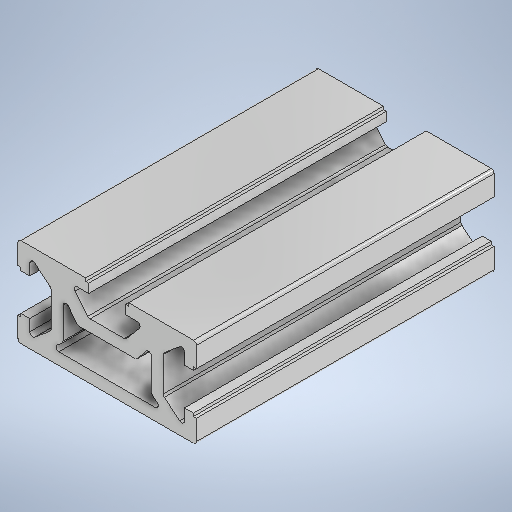
# Autodesk Inventor part: perfil_15x30_001
Saved by Autodesk Inventor 2025.2 (Build 292293000, 293)
## iProperties
Created: 2025-03-25
Part Number: perfil_15x30_001
Material: Alumínio 6061
Document SubType Name: Modeling
Designer: Carlos Dias
Density: 2.7 g/cm^3
Appearance: Alumínio - Polido
Author: Carlos Dias
Autodesk Inventor part; units mm, degrees
ref_plane "YZ Plane" through (0, 0, 0) normal (1, 0, 0) x (0, 1, 0)
ref_plane "XZ Plane" through (0, 0, 0) normal (0, 1, 0) x (-1, 0, 0)
ref_plane "XY Plane" through (0, 0, 0) normal (0, 0, 1) x (1, 0, 0)
sketch "Esboço1" plane through (0, 0, 0) normal (0, 0, 1) x (1, 0, 0)
  line L0 (-15, 15) -> (15, 15) construction
  line L1 (-15, 15) -> (-15, 10.6) construction
  line L2 (-15, 10.6) -> (-13, 10.6) construction
  line L3 (-13, 13.6) -> (-13, 10.6) construction
  line L4 (-13, 13.6) -> (-9.4247, 10.6) construction
  line L5 (-9.4247, 10.6) -> (-9.4247, 4.4) construction
  line L6 (-9.4247, 4.4) -> (-13, 1.4) construction
  line L7 (-13, 4.4) -> (-13, 1.4) construction
  line L8 (-15, 4.4) -> (-13, 4.4) construction
  line L9 (-15, 4.4) -> (-15, 0) construction
  line L10 (-15, 0) -> (0, 0) construction
  line L11 (-15, 4.4) -> (-14.5, 4.4) construction
  line L12 (-14.5, 4.4) -> (-14.5, 3.9)
  line L13 (-14.5, 3.9) -> (-15, 3.9)
  line L14 (-15, 3.9) -> (-15, 4.4) construction
  line L15 (-15, 10.6) -> (-14.5, 10.6) construction
  line L16 (-14.5, 10.6) -> (-14.5, 11.1)
  line L17 (-14.5, 11.1) -> (-15, 11.1)
  line L18 (-15, 11.1) -> (-15, 10.6) construction
  line L19 (-3.1, 9.4247) -> (3.1, 9.4247) construction
  line L20 (-6.1, 13) -> (-3.1, 9.4247) construction
  line L21 (-6.1, 13) -> (-3.1, 13) construction
  line L22 (-3.1, 15) -> (-3.1, 13) construction
  line L23 (-3.1, 9.4247) -> (0, 9.4247) construction
  line L24 (-3.1, 15) -> (-3.6, 15) construction
  line L25 (-3.6, 15) -> (-3.6, 14.5)
  line L26 (-3.6, 14.5) -> (-3.1, 14.5)
  line L27 (-3.1, 14.5) -> (-3.1, 15) construction
  line L28 (-9.4247, 2) -> (0, 2) construction
  line L29 (-7.4247, 3.6782) -> (-9.4247, 2) construction
  line L30 (-7.4247, 10.6) -> (-7.4247, 3.6782) construction
  line L31 (-7.4247, 10.6) -> (-4.944, 7.4247) construction
  line L32 (-4.944, 7.4247) -> (0, 7.4247) construction
  arc A0 (-14.5, 15) -> (-15, 14.5) centre (-14.5, 14.5) ccw
  arc A1 (-12.1786, 12.9108) -> (-13, 12.5277) centre (-12.5, 12.5277) ccw
  line L33 (-14.5, 15) -> (-3.6, 15)
  line L34 (-13, 12.5277) -> (-13, 10.6)
  line L35 (-13, 10.6) -> (-14.5, 10.6)
  arc A2 (-9.4247, 10.3668) -> (-9.6033, 10.7499) centre (-9.9247, 10.3668) ccw
  arc A3 (-9.6033, 4.2501) -> (-9.4247, 4.6332) centre (-9.9247, 4.6332) ccw
  arc A4 (-13, 2.4723) -> (-12.1786, 2.0892) centre (-12.5, 2.4723) ccw
  line L36 (-12.1786, 12.9108) -> (-9.6033, 10.7499)
  line L37 (-9.4247, 10.3668) -> (-9.4247, 4.6332)
  line L38 (-9.6033, 4.2501) -> (-12.1786, 2.0892)
  line L39 (-13, 2.4723) -> (-13, 4.4)
  arc A5 (-15, 0.5) -> (-14.5, 0) centre (-14.5, 0.5) ccw
  line L40 (-15, 14.5) -> (-15, 11.1)
  line L41 (-15, 3.9) -> (-15, 0.5)
  line L42 (-14.5, 0) -> (0, 0)
  arc A6 (-8.4247, 2.8391) -> (-8.1193, 2) centre (-8.1193, 2.4751) ccw
  arc A7 (-6.5307, 9.4557) -> (-7.4247, 9.1479) centre (-6.9247, 9.1479) ccw
  line L43 (-8.1193, 2) -> (0, 2)
  arc A8 (-7.6033, 3.5283) -> (-7.4247, 3.9114) centre (-7.9247, 3.9114) ccw
  arc A9 (-5.0941, 7.6169) -> (-4.7001, 7.4247) centre (-4.7001, 7.9247) ccw
  arc A10 (-3.2499, 9.6033) -> (-2.8668, 9.4247) centre (-2.8668, 9.9247) ccw
  arc A11 (-5.0277, 13) -> (-5.4108, 12.1786) centre (-5.0277, 12.5) ccw
  line L44 (-5.0277, 13) -> (-3.1, 13)
  line L45 (-5.4108, 12.1786) -> (-3.2499, 9.6033)
  line L46 (-2.8668, 9.4247) -> (0, 9.4247)
  line L47 (-4.7001, 7.4247) -> (0, 7.4247)
  line L48 (-6.5307, 9.4557) -> (-5.0941, 7.6169)
  line L49 (-7.4247, 9.1479) -> (-7.4247, 3.9114)
  line L50 (0, 2) -> (0, 0)
  line L51 (0, 7.4247) -> (0, 9.4247)
  line L52 (-3.1, 14.5) -> (-3.1, 13)
  line L53 (-14.5, 4.4) -> (-13, 4.4)
  line L54 (-8.4247, 2.8391) -> (-7.6033, 3.5283)
  point P0 (0, 0)
  point P1 (0, 15)
  point P2 (-14, 4.4)
  point P3 (-1.55, 9.4247)
  point P4 (-9.6033, 10.7499)
  dimension "d0" = 30
  dimension "d1" = 15
  dimension "d6" = 2
  dimension "d7" = 3
  dimension "d9" = 50
  dimension "d12" = 0.5
  dimension "d18" = 50
  dimension "d19" = 2
  dimension "d21" = 2
  dimension "d22" = 2
  dimension "d24" = 2
  dimension "d25" = 0.5
  dimension "d26" = 0.5
  dimension "d27" = 0.5
  dimension "d28" = 0.5
  dimension "d29" = 0.5
  dimension "d30" = 0.5
  dimension "d31" = 0.5
  dimension "d32" = 0.5
  dimension "d33" = 0.5
  dimension "d34" = 0.5
  dimension "d35" = 0.5
  dimension "d38" = 3.1
  dimension "d39" = 6.2
  dimension "d40" = 15
  constraints: 110 end point, 29 point on line, 27 tangent, 24 point on circle, 16 collinear, 12 centre point, 12 equal length, 12 horizontal, 9 vertical, 7 parallel, 7 vertical alignment, 5 midpoint, 4 perpendicular, 2 horizontal alignment, 1 coincident
  measures "d0" distance of L0.start L0.end
  measures "d1" distance from line of point (0, 0) L0
  measures "d6" distance of L1.end L2.end
  measures "d7" distance of L3.start L2.end
  measures "d9" angle of L4 L3
  measures "d12" distance of L16.end L17.end
  measures "d18" angle of L20 L21
  measures "d19" distance between parallel lines of L10 L28
  measures "d21" distance between parallel lines of L5 L30
  measures "d22" angle of L20 L31
  measures "d24" distance between parallel lines of L19 L32
  measures "d25" radius of A0
  measures "d26" radius of A2
  measures "d27" radius of A3
  measures "d28" radius of A4
  measures "d29" radius of A1
  measures "d30" radius of A5
  measures "d31" radius of A8
  measures "d32" radius of A9
  measures "d33" radius of A10
  measures "d34" radius of A11
  measures "d35" radius of A7
  measures "d38" horizontal distance of point (0, 0) L22.start
  measures "d39" distance of L8.start L1.end
  measures "d40" distance between parallel lines of L10 L0
extrude "Extrusão1" add sketch "Esboço1" along normal mid plane 50
mirror "Espelhar1" about plane through (0, 0, 0) normal (1, 0, 0) of "Extrusão1"
equation "\"d6\" = d21"
equation "\"d18\" = d9"
equation "\"d19\" = d21"
equation "\"d22\" = d20"
equation "\"d24\" = d21"
equation "\"d25\" = d35"
equation "\"d26\" = d35"
equation "\"d27\" = d35"
equation "\"d28\" = d35"
equation "\"d29\" = d35"
equation "\"d30\" = d35"
equation "\"d31\" = d35"
equation "\"d32\" = d35"
equation "\"d33\" = d35"
equation "\"d34\" = d35"
equation "\"d39\" = 2 * d38"
equation "\"d20\" = 2deg"
